bracket joint (Autodesk Fusion 360 design; units mm, degrees)
Autodesk Fusion 360 part; units mm, degrees
note: some values were not read from the file. Set by a fixed rule: which sketch regions a step uses.
sketch "Sketch1" plane through (0, 0, 0) normal (0, 1, 0) x (1, 0, 0) in component "Component"
  line L0 (0, 0) -> (40, 0)
  line L1 (40, 0) -> (40, -40)
  line L2 (40, -40) -> (0, -40)
  line L3 (0, -40) -> (0, 0)
  line L4 (0, -40) -> (40, 0)
  dimension "d1" = 40
  constraint horizontal L0
  constraint vertical L1
  constraint horizontal L2
  constraint vertical L3
  constraint coincident L0.start L3.end
  measures "d1" distance of L0.start L0.end
sketch "Sketch2" plane through (0, 0, 0) normal (0, 0, 1) x (1, 0, 0) in component "Component"
  line L0 (0, 0) -> (40, 0)
  line L1 (40, 0) -> (40, 40)
  line L2 (40, 40) -> (0, 40)
  line L3 (0, 40) -> (0, 0)
  line L4 (0, 40) -> (40, 0)
  circle A0 centre (10, 10) radius 1.5
  dimension "d4" = 3
  constraint horizontal L0
  constraint vertical L1
  constraint horizontal L2
  constraint vertical L3
  constraint coincident L0.start L3.end
  measures "d4" diameter of A0
sketch "Sketch3" plane through (0, 0, 0) normal (1, 0, 0) x (0, 0, -1) in component "Component"
  line L0 (0, 0) -> (-40, 0)
  line L1 (-40, 0) -> (-40, 40)
  line L2 (-40, 40) -> (0, 40)
  line L3 (0, 40) -> (0, 0)
  constraint horizontal L0
  constraint vertical L1
  constraint horizontal L2
  constraint vertical L3
  constraint coincident L0.start L3.end
sketch "Sketch4" plane through (0, 0, 0) normal (1, 0, 0) x (0, 0, -1) in component "Component"
  line L0 (-40, 0) -> (0, 0)
  line L1 (0, 0) -> (0, 40)
  line L2 (0, 40) -> (-40, 40)
  line L3 (-40, 40) -> (-40, 0)
  line L4 (-40, 0) -> (0, 40)
  point P0 (-40, 0)
  point P1 (0, 40)
  constraint horizontal L0
  constraint vertical L1
  constraint horizontal L2
  constraint vertical L3
  constraint coincident P1 L1.end
  constraint coincident P0 L0.start
sketch "Sketch5" plane through (0, 0, 0) normal (1, 0, 0) x (0, 0, -1) in component "Component"
  line L0 (0, 40) -> (0, 0)
  circle A0 centre (-10, 10) radius 1.5
  point P0 (-40, 40)
  dimension "d3" = 3
  measures "d3" diameter of A0
sketch "Sketch6" plane through (0, 0, 0) normal (0, 1, 0) x (1, 0, 0) in component "Component"
  line L0 (0, 0) -> (40, -40)
  line L1 (0, 0) -> (0, -40)
  circle A0 centre (10, -10) radius 1.5
  point P0 (40, -40)
  dimension "d2" = 3
  constraint coincident L0.start L1.start
  constraint coincident P0 L0.end
  measures "d2" diameter of A0
extrude "Extrude1" add sketch "Sketch3" against normal blind 5 makes body 1 in component "Component"
extrude "Extrude2" add sketch "Sketch2" against normal blind 5 separate body contours L0 L3 L4 makes body 2 in component "Component"
extrude "Extrude3" cut sketch "Sketch4" against normal blind 12 contours L2 L3 L4 bodies 1 in component "Component"
extrude "Extrude4" cut sketch "Sketch5" against normal blind 9 bodies 1 in component "Component"
extrude "Extrude5" add sketch "Sketch1" against normal blind 5 separate body contours L0 L3 L4 makes body 3 in component "Component"
extrude "Extrude6" cut sketch "Sketch6" against normal blind 31 bodies 3 in component "Component"
sketch "Sketch7" plane through (0, 0, 0) normal (0, 0, -1) x (-1, 0, 0) in component "Component"
  line L0 (0, 0) -> (-40, 0)
  line L1 (-40, 0) -> (-40, -5)
  line L2 (-40, -5) -> (0, -5)
  line L3 (0, -5) -> (0, 0)
  line L4 (0, -5) -> (5, 0)
  line L5 (5, 0) -> (0, 0)
  line L6 (0, -5) -> (0, 0)
  line L7 (5, 0) -> (0, 0)
  constraint coincident L2.end L3.start
  constraint coincident L0.start L3.end
  constraint perpendicular L3 L5
extrude "Extrude7" add sketch "Sketch7" against normal blind 40 contours L3 L4 L5 L6 L7 bodies 1 2 3 in component "Component"
sketch "Sketch8" plane through (0, 0, 0) normal (0, -1, 0) x (1, 0, 0) in component "Component"
  line L0 (40, 0) -> (0, 0)
  line L1 (0, 0) -> (0, -5)
  line L2 (0, -5) -> (40, -5)
  line L3 (40, -5) -> (40, 0)
  line L4 (-5, 0) -> (0, -5)
  line L5 (0, 0) -> (-5, 0)
  line L6 (0, -5) -> (0, 0)
  point P0 (-5, 0)
  point P1 (-5, 0)
  constraint coincident P1 P0
  constraint coincident L1.end L2.start
  constraint coincident L0.end L1.start
extrude "Extrude8" add sketch "Sketch8" against normal blind 40 separate body contours L1 L4 L5 L6 makes body 4 in component "Component"
sketch "Sketch9" plane through (0, 0, 0) normal (1, 0, 0) x (0, 0, -1) in component "Component"
  line L0 (0, 0) -> (0, -5)
  line L1 (0, 0) -> (0, -5)
  line L2 (5, 0) -> (0, 0)
  line L3 (0, -5) -> (5, 0)
  point P0 (0, -5)
  point P1 (5, 0)
  constraint coincident L0.start L1.start
  constraint coincident P0 L0.end
  constraint coincident P1 L2.start
extrude "Extrude9" add sketch "Sketch9" along normal blind 40 separate body makes body 5 in component "Component"
move_face "OffsetFaces1" offset 5 1 faces at (-1.6667, 0, -1.6667) on bodies 4 in component "Component"
sketch "Sketch10" plane through (0, 0, 0) normal (0, 0, 1) x (1, 0, 0) in component "Component"
  line L0 (-5, -5) -> (0, -5)
  line L1 (0, -5) -> (0, 40)
  line L2 (0, 40) -> (-5, 40)
  line L3 (-5, 40) -> (-5, -5)
  line L4 (-5, 0.0489) -> (0, -5)
  line L5 (-5, -5) -> (-5, 0.0489)
  constraint coincident L3 L4.start
  constraint coincident L0.end L1.start
  constraint coincident L0.start L3.end
extrude "Extrude10" cut sketch "Sketch10" against normal blind 17 contours L0 L3 L4 L5 bodies 4 in component "Component"
sketch "Sketch11" plane through (0, 0, 0) normal (1, 0, 0) x (0, 0, -1) in component "Component"
  line L0 (0, -5) -> (5, -5)
  line L1 (5, -5) -> (5, 40)
  line L2 (5, 40) -> (0, 40)
  line L3 (0, 40) -> (0, -5)
  line L4 (0, -5) -> (5, 0)
  line L5 (5, -5) -> (0, -5)
  line L6 (5, 0) -> (5, -5)
  point P0 (5, 0)
  constraint coincident L0.start L3.end
  constraint coincident P0 L4.end
  constraint coincident L0.end L1.start
extrude "Extrude11" cut sketch "Sketch11" against normal blind 18 contours L0 L1 L4 L5 L6 bodies 4 in component "Component"
sketch "Sketch12" plane through (0, 0, 0) normal (0, 1, 0) x (1, 0, 0) in component "Component"
  line L0 (47, 2) -> (47, -47)
  line L1 (47, -47) -> (-2, -47)
  line L2 (-2, -47) -> (-2, 2)
  line L3 (-2, 2) -> (47, 2)
extrude "Extrude12" cut sketch "Sketch12" along normal blind 65 bodies 1 4 makes body 6 at (17.0332, 0, 17.0068) in component "Component"
extrude "Extrude13" cut sketch "Sketch12" against normal blind 2 bodies 4 5 6 in component "Component"
sketch "Sketch13" plane through (0, 0, -5) normal (0, 0, -1) x (-1, 0, 0) in component "Component"
  circle A0 centre (-10, 10) radius 1.5
  line L0 (-40, 0) -> (0, 0)
  line L1 (0, 0) -> (0, 40)
  line L2 (0, 40) -> (-40, 0)
  circle A1 centre (-10, 10) radius 3.5
  dimension "d33" = 7
  constraint concentric A0 A1
  measures "d33" diameter of A1
extrude "Extrude14" cut sketch "Sketch13" against normal blind 1 contours A1 bodies 1 in component "Component"
sketch "Sketch14" plane through (-5, 0, 0) normal (-1, 0, 0) x (0, 0, 1) in component "Component"
  circle A0 centre (10, 10) radius 1.5
  line L0 (40, 0) -> (0, 40)
  line L1 (0, 40) -> (0, 0)
  line L2 (0, 0) -> (40, 0)
  circle A1 centre (10, 10) radius 3.5
  dimension "d36" = 7
  constraint concentric A0 A1
  measures "d36" diameter of A1
extrude "Extrude15" cut sketch "Sketch14" against normal blind 1 contours A1 bodies 6 in component "Component"
sketch "Sketch15" plane through (0, -5, 0) normal (0, -1, 0) x (1, 0, 0) in component "Component"
  circle A0 centre (10, 10) radius 1.5
  line L0 (0, 40) -> (0, 0)
  line L1 (0, 0) -> (40, 0)
  line L2 (40, 0) -> (0, 40)
  circle A1 centre (10, 10) radius 3.5
  dimension "d39" = 7
  constraint concentric A0 A1
  measures "d39" diameter of A1
extrude "Extrude16" cut sketch "Sketch15" against normal blind 1 contours A1 bodies 6 in component "Component"
sketch "Sketch16" plane through (40, 0, 0) normal (1, 0, 0) x (0, 0, -1) in component "Component"
  line L0 (2, 0) -> (2, -2)
  line L1 (2, -2) -> (0, -2)
  line L2 (0, -2) -> (0, -5)
  line L3 (0, -5) -> (5, 0)
  line L4 (5, 0) -> (2, 0)
  line L5 (0, -5) -> (5, -5)
  line L6 (5, -5) -> (5, 0)
  constraint coincident L2.end L3.start
  constraint perpendicular L2 L5
  constraint coincident L3.end L4.start
extrude "Extrude17" add sketch "Sketch16" against normal blind 40 contours L3 L5 L6 bodies 5 1 4 6 in component "Component"
sketch "Sketch17" plane through (0, 0, 40) normal (0, 0, 1) x (1, 0, 0) in component "Component"
  line L0 (0, -2) -> (-2, -2)
  line L1 (-2, -2) -> (-2, 0)
  line L2 (-2, 0) -> (-5, 0)
  line L3 (-5, 0) -> (0, -5)
  line L4 (0, -5) -> (0, -2)
  line L5 (-5, 0) -> (0, -5)
  line L6 (-5, -5) -> (-5, 0)
  line L7 (0, -5) -> (-5, -5)
  constraint coincident L2.end L3.start
  constraint coincident L3.end L4.start
  constraint perpendicular L2 L6
  constraint perpendicular L6 L7
extrude "Extrude18" add sketch "Sketch17" against normal blind 40 contours L3 L5 L6 L7 bodies 5 in component "Component"
sketch "Sketch18" plane through (0, 40, 0) normal (0, 1, 0) x (-1, 0, 0) in component "Component"
  line L0 (2, -2) -> (0, -2)
  line L1 (0, -2) -> (0, -5)
  line L2 (0, -5) -> (5, 0)
  line L3 (5, 0) -> (2, 0)
  line L4 (2, 0) -> (2, -2)
  line L5 (5, 0) -> (5, -5)
  line L6 (5, -5) -> (0, -5)
  line L7 (5, 0) -> (0, -5)
  constraint coincident L2.end L3.start
  constraint perpendicular L3 L5
  constraint coincident L1.end L2.start
extrude "Extrude19" add sketch "Sketch18" against normal blind 45 separate body contours L2 L5 L6 L7 makes body 7 in component "Component"
sketch "Sketch19" plane through (0, -5, 0) normal (0, -1, 0) x (1, 0, 0) in component "Component"
  line L0 (-5, 0) -> (-5, -5)
  line L1 (-5, -5) -> (0, -5)
  line L2 (0, -5) -> (-5, 0)
  line L3 (-5, 0) -> (0, 0)
  line L4 (0, 0) -> (0, -5)
  line L5 (0, -5) -> (-5, -5)
  line L6 (-5, -5) -> (-5, 0)
  constraint horizontal L3
  constraint vertical L4
  constraint horizontal L5
  constraint vertical L6
  constraint coincident L1.end L2.start
  constraint coincident L0.start L2.end
extrude "Extrude20" add sketch "Sketch19" against normal blind 3 contours L2 L3 L4 bodies 5 7 in component "Component"
component "Component" placed x (1, 0, 0) y (0, 1, 0) z (0, 0, 1) at (15.4578, -1.4684, -4.3289)
